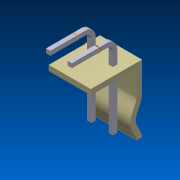
# Autodesk Inventor part: conn_sensor
Saved by Autodesk Inventor 2015 SP1 (Build 190203100, 203)
## iProperties
Created: 2015-12-01
Part Number: conn_sensor
Material: Generic
Document SubType Name: Modeling
Designer: User
Density: 1 g/cm^3
Appearance: Default
Author: User
Autodesk Inventor part; units mm, degrees
ref_plane "YZ Plane" through (0, 0, 0) normal (1, 0, 0) x (0, 1, 0)
ref_plane "XY Plane" through (0, 0, 0) normal (0, 0, 1) x (1, 0, 0)
sketch "Эскиз1" plane through (0, 0, 0) normal (1, 0, 0) x (0, 1, 0)
  line L0 (-3, -4.5) -> (6, -4.5)
  line L1 (0, -19.9641) -> (0, 3.794) projected
  line L2 (-7.2118, 0) -> (8.271, 0) projected
  line L3 (6, -4.5) -> (6, -9.5)
  line L4 (6, -9.5) -> (6, -11.6158) construction
  line L5 (6, -11.6158) -> (2.9383, -13.3469) construction
  line L6 (2.9383, -13.3469) -> (6, -14.7108) construction
  line L7 (6, -14.7108) -> (6, -16.5) construction
  spline S0 degree 4 poles (6, -9.5) (6, -11.6158) (2.9383, -13.3469) (6, -14.7108) (6, -16.5) knots 1 1 1 1 1 2 2 2 2 2
  line L8 (-5, 0) -> (1.5, 0)
  line L9 (3, -1.5) -> (3, -15)
  arc A0 (3, -1.5) -> (1.5, 0) centre (1.5, -1.5) ccw
  point P0 (0, 0)
  dimension "d0" = 9
  dimension "d1" = 3
  dimension "d2" = 4.5
  dimension "d3" = 5
  dimension "d4" = 12
  dimension "d5" = 7
  dimension "d7" = 3
  dimension "d9" = 3
  dimension "d11" = 15
  dimension "d12" = 8
  constraints: 8 end point, 2 horizontal, 2 point on circle, 2 point on line, 2 tangent, 2 vertical, 1 centre point, 1 perpendicular, 3 other
  measures "d0" distance of L0.start L0.end
  measures "d1" distance from line of L1 L0.start
  measures "d2" distance between parallel lines of L2 L0
  measures "d3" distance of L0.end L3.end
  measures "d4" distance of L0.end L7.end
  measures "d5" distance of L7.end L3.end
  measures "d7" diameter of A0
  measures "d9" distance between parallel lines of L1 L9
  measures "d11" distance from line of L8 L9.end
  measures "d12" distance from line of L9 L8.start
ref_plane "РабПлоскость1" through (0, -5, 0) normal (0, 1, 0) x (-1, 0, 0)
ref_plane "РабПлоскость2" through (0, -3, 0) normal (0, 1, 0) x (-1, 0, 0)
sketch "Эскиз2" plane through (0, -3, 0) normal (0, 1, 0) x (-1, 0, 0)
  line L0 (-3.9, -4) -> (3.9, -4)
  line L1 (3.9, -4) -> (3.9, -5)
  line L2 (3.9, -5) -> (-3.9, -5)
  line L3 (-3.9, -5) -> (-3.9, -4)
  line L4 (0, -5.48) -> (0, 1.38) projected
  line L5 (0, -4.5) -> (1.03, -4.5)
  point P0 (0, 0)
  dimension "d15" = 7.8
  dimension "d16" = 1
  constraints: 10 end point, 2 horizontal, 2 parallel, 1 perpendicular, 2 other
  measures "d15" distance of L1.end L2.end
  measures "d16" distance of L0.end L1.end
sweep "Сдвиг1" add profiles "Эскиз2" path "Эскиз1" path curves L0 L3 S0
sketch "Эскиз3" plane through (0, -5, 0) normal (0, 1, 0) x (-1, 0, 0)
  line L0 (3.36, 0) -> (-3.36, 0) projected
  line L1 (0, -0.56) -> (0, 0.56) projected
  line L2 (2.4, 0.4) -> (1.6, 0.4)
  line L3 (1.6, 0.4) -> (1.6, -0.4)
  line L4 (1.6, -0.4) -> (2.4, -0.4)
  line L5 (2.4, -0.4) -> (2.4, 0.4)
  line L6 (-1.6, 0.4) -> (-2.4, 0.4)
  line L7 (-2.4, 0.4) -> (-2.4, -0.4)
  line L8 (-2.4, -0.4) -> (-1.6, -0.4)
  line L9 (-1.6, -0.4) -> (-1.6, 0.4)
  point P0 (0, 0)
  dimension "d22" = 0.8
  dimension "d23" = 0.8
  dimension "d24" = 0.8
  dimension "d25" = 0.8
  dimension "d26" = 4
  constraints: 16 end point, 4 parallel, 2 horizontal, 2 perpendicular, 3 other
  measures "d22" distance of L4.end L3.end
  measures "d23" distance of L3.end L2.end
  measures "d24" distance of L8.end L7.end
  measures "d25" distance of L7.end L6.end
  measures "d26" distance between parallel lines of L7 L3
sweep "Сдвиг2" add profiles "Эскиз3" path "Эскиз1" path curves L8 A0 L9
sketch "Эскиз4" plane through (0, 0, 0) normal (0, 1, 0) x (-1, 0, 0)
  line L0 (2.4, 0.4) -> (1.6, 0.4) projected
  line L1 (2.4, -0.4) -> (2.4, 0.4) projected
  line L2 (1.6, -0.4) -> (2.4, -0.4) projected
  line L3 (1.6, 0.4) -> (1.6, -0.4) projected
  line L4 (-1.6, 0.4) -> (-2.4, 0.4) projected
  line L5 (-1.6, -0.4) -> (-1.6, 0.4) projected
  line L6 (-2.4, -0.4) -> (-1.6, -0.4) projected
  line L7 (-2.4, 0.4) -> (-2.4, -0.4) projected
  line L8 (2.4, 0.4) -> (1.6, 0.4) projected
  line L9 (1.6, 0.4) -> (1.6, -0.4) projected
  line L10 (1.6, -0.4) -> (2.4, -0.4) projected
  line L11 (2.4, -0.4) -> (2.4, 0.4) projected
  line L12 (-2.4, -0.4) -> (-1.6, -0.4) projected
  line L13 (-1.6, -0.4) -> (-1.6, 0.4) projected
  line L14 (-1.6, 0.4) -> (-2.4, 0.4) projected
  line L15 (-2.4, 0.4) -> (-2.4, -0.4) projected
  circle A0 centre (-2, 0) radius 0.5657
  point P0 (0, 0)
  constraints: 3 point on circle, 1 centre point
